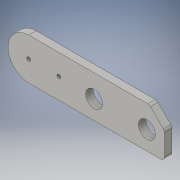
# Autodesk Inventor part: Top IntakeBar
Saved by Autodesk Inventor 2016 (Build 200138000, 138)
## iProperties
Created: 2016-01-16
Part Number: Top IntakeBar
Material: Generic
Document SubType Name: Modeling
Designer: Mentor1102
Density: 1 g/cm^3
Appearance: Default
Author: Mentor1102
Autodesk Inventor part; units mm, degrees
ref_plane "YZ Plane" through (0, 0, 0) normal (1, 0, 0) x (0, 1, 0)
ref_plane "XZ Plane" through (0, 0, 0) normal (0, 1, 0) x (-1, 0, 0)
ref_plane "XY Plane" through (0, 0, 0) normal (0, 0, 1) x (1, 0, 0)
sketch "Sketch1" plane through (0, 0, 0) normal (0, 0, 1) x (1, 0, 0)
  line L0 (90.332, 117.5659) -> (90.332, 153.0357)
  line L1 (88.4722, 157.5258) -> (66.7919, 179.2061)
  line L2 (62.3018, 181.0659) -> (-138.268, 181.0659)
  circle A0 centre (60.8045, 142.9659) radius 14.2875
  arc A1 (66.7919, 179.2061) -> (62.3018, 181.0659) centre (62.3018, 174.7159) ccw
  arc A2 (90.332, 153.0357) -> (88.4722, 157.5258) centre (83.982, 153.0357) ccw
  arc A3 (83.982, 111.2159) -> (90.332, 117.5659) centre (83.982, 117.5659) ccw
  line L3 (-138.268, 111.2159) -> (83.982, 111.2159)
  arc A4 (-138.268, 181.0659) -> (-138.268, 111.2159) centre (-138.268, 146.1409) ccw
  circle A5 centre (-138.268, 146.1409) radius 3.175
  dimension "d61" = 69.85
  dimension "d68" = 222.25
  dimension "d69" = 200.5697
  dimension "d71" = 28.575
  dimension "d72" = 6.35
  constraints: 8 end point, 8 point on circle, 7 tangent, 6 centre point, 1 coincident, 1 horizontal, 1 parallel
  measures "d61" distance between parallel lines of L3 L2
  measures "d68" distance of L3.start L3.end
  measures "d69" distance of L2.start L2.end
  measures "d71" diameter of A0
  measures "d72" diameter of A5
extrude "Extrusion10" add sketch "Sketch1" along normal blind 12.7
sketch "Sketch8" plane through (0, 0, 12.7) normal (0, 0, 1) x (1, 0, 0)
  circle A0 centre (60.8045, 142.9659) radius 14.2875 projected
  circle A1 centre (-138.268, 146.1409) radius 3.175 projected
  line L0 (62.3018, 181.0659) -> (-138.268, 181.0659) projected
  arc A2 (-138.268, 181.0659) -> (-138.268, 111.2159) centre (-138.268, 146.1409) ccw projected
  line L1 (-138.268, 111.2159) -> (83.982, 111.2159) projected
  arc A3 (83.982, 111.2159) -> (90.332, 117.5659) centre (83.982, 117.5659) ccw projected
  line L2 (90.332, 117.5659) -> (90.332, 153.0357) projected
  arc A4 (90.332, 153.0357) -> (88.4722, 157.5258) centre (83.982, 153.0357) ccw projected
  line L3 (88.4722, 157.5258) -> (66.7919, 179.2061) projected
  arc A5 (66.7919, 179.2061) -> (62.3018, 181.0659) centre (62.3018, 174.7159) ccw projected
  circle A6 centre (60.8045, 142.9659) radius 50.8 construction
  line L4 (60.8045, 142.9659) -> (-28.0955, 142.9659) construction
  circle A7 centre (-28.0955, 142.9659) radius 14.2875
  point P0 (0, 0)
  dimension "d75" = 101.6
  dimension "d76" = 88.9
  dimension "d77" = 28.575
  constraints: 2 centre point, 2 coincident, 2 end point, 1 horizontal
  measures "d75" diameter of A6
  measures "d76" distance of L4.start L4.end
  measures "d77" diameter of A7
extrude "Extrusion11" cut sketch "Sketch8" against normal through all contours A7
sketch "Sketch9" plane through (0, 0, 12.7) normal (0, 0, 1) x (1, 0, 0)
  circle A0 centre (-28.0955, 142.9659) radius 14.2875 projected
  circle A1 centre (60.8045, 142.9659) radius 14.2875 projected
  circle A2 centre (-138.268, 146.1409) radius 3.175 projected
  line L0 (62.3018, 181.0659) -> (-138.268, 181.0659) projected
  arc A3 (-138.268, 181.0659) -> (-138.268, 111.2159) centre (-138.268, 146.1409) ccw projected
  line L1 (-138.268, 111.2159) -> (83.982, 111.2159) projected
  arc A4 (83.982, 111.2159) -> (90.332, 117.5659) centre (83.982, 117.5659) ccw projected
  line L2 (90.332, 117.5659) -> (90.332, 153.0357) projected
  arc A5 (90.332, 153.0357) -> (88.4722, 157.5258) centre (83.982, 153.0357) ccw projected
  line L3 (88.4722, 157.5258) -> (66.7919, 179.2061) projected
  arc A6 (66.7919, 179.2061) -> (62.3018, 181.0659) centre (62.3018, 174.7159) ccw projected
  line L4 (60.8045, 142.9659) -> (111.6045, 142.9659)
  line L5 (-173.193, 146.1409) -> (-173.193, 114.3909)
  line L6 (60.8045, 142.9659) -> (-173.193, 142.9659)
  point P0 (0, 0)
  dimension "d80" = 50.8
  dimension "d81" = 284.7975
  constraints: 6 end point, 1 horizontal, 1 perpendicular, 1 point on circle, 1 point on line, 1 vertical
  measures "d80" distance of L4.start L4.end
  measures "d81" distance of L6.end L4.end
sketch "Sketch10" plane through (0, 0, 12.7) normal (0, 0, 1) x (1, 0, 0)
  circle A0 centre (-28.0955, 142.9659) radius 14.2875 projected
  circle A1 centre (60.8045, 142.9659) radius 14.2875 projected
  circle A2 centre (-138.268, 146.1409) radius 3.175 projected
  line L0 (62.3018, 181.0659) -> (-138.268, 181.0659) projected
  arc A3 (-138.268, 181.0659) -> (-138.268, 111.2159) centre (-138.268, 146.1409) ccw projected
  line L1 (-138.268, 111.2159) -> (83.982, 111.2159) projected
  arc A4 (83.982, 111.2159) -> (90.332, 117.5659) centre (83.982, 117.5659) ccw projected
  line L2 (90.332, 117.5659) -> (90.332, 153.0357) projected
  arc A5 (90.332, 153.0357) -> (88.4722, 157.5258) centre (83.982, 153.0357) ccw projected
  line L3 (88.4722, 157.5258) -> (66.7919, 179.2061) projected
  arc A6 (66.7919, 179.2061) -> (62.3018, 181.0659) centre (62.3018, 174.7159) ccw projected
  line L4 (-138.268, 146.1409) -> (-87.468, 146.1409) construction
  circle A7 centre (-87.468, 146.1409) radius 3.175
  point P0 (0, 0)
  dimension "d82" = 50.8
  dimension "d83" = 6.35
  constraints: 2 end point, 1 centre point, 1 coincident, 1 horizontal
  measures "d82" distance of L4.start L4.end
  measures "d83" diameter of A7
extrude "Extrusion12" cut sketch "Sketch10" against normal through all contours A7
body "Solid6"
